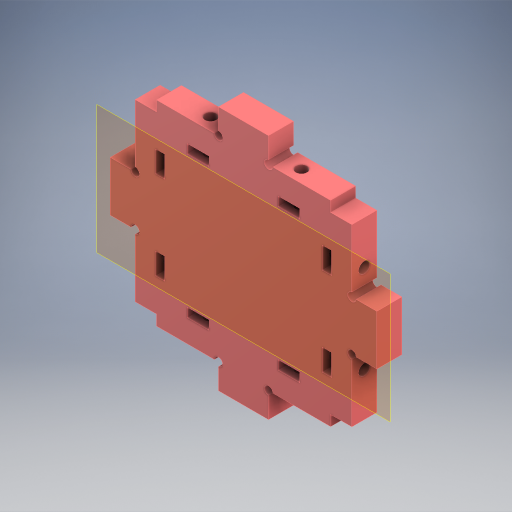
# Autodesk Inventor part: connection_leg_ver2
Saved by Autodesk Inventor 2024 (Build 280153000, 153)
## iProperties
Created: 2024-09-05
Part Number: connection_leg_ver2
Material: PMMA 플라스틱
Document SubType Name: Modeling
Designer: msi
Density: 1.188 g/cm^3
Appearance: 매끄러움 - 빨간색
Author: msi
Autodesk Inventor part; units mm, degrees
ref_plane "YZ Plane" through (0, 0, 0) normal (1, 0, 0) x (0, 1, 0)
ref_plane "XZ Plane" through (0, 0, 0) normal (0, 1, 0) x (-1, 0, 0)
ref_plane "XY Plane" through (0, 0, 0) normal (0, 0, 1) x (1, 0, 0)
ref_plane "작업 평면1" through (0, 0, 0) normal (0, 0, 1) x (1, 0, 0)
sketch "스케치1" plane through (0, 0, 0) normal (0, 0, 1) x (1, 0, 0)
  line L0 (-18.9, 5.4) -> (-21.1, 5.4) projected
  line L1 (-21.1, 5.4) -> (-21.1, 10.6) projected
  line L2 (-21.1, 10.6) -> (-18.9, 10.6) projected
  line L3 (-18.9, 10.6) -> (-18.9, 5.4) projected
  line L4 (-21.1, -5.4) -> (-18.9, -5.4) projected
  line L5 (-18.9, -5.4) -> (-18.9, -10.6) projected
  line L6 (-18.9, -10.6) -> (-21.1, -10.6) projected
  line L7 (-21.1, -10.6) -> (-21.1, -5.4) projected
  line L8 (21.1, 5.4) -> (18.9, 5.4) projected
  line L9 (18.9, 5.4) -> (18.9, 10.6) projected
  line L10 (18.9, 10.6) -> (21.1, 10.6) projected
  line L11 (21.1, 10.6) -> (21.1, 5.4) projected
  line L12 (18.9, -10.6) -> (18.9, -5.4) projected
  line L13 (18.9, -5.4) -> (21.1, -5.4) projected
  line L14 (21.1, -5.4) -> (21.1, -10.6) projected
  line L15 (21.1, -10.6) -> (18.9, -10.6) projected
  circle A0 centre (8, -8) radius 1.35 projected
  circle A1 centre (-8, 8) radius 1.35 projected
  circle A2 centre (-8, -8) radius 1.35 projected
  circle A3 centre (8, 8) radius 1.35 projected
  line L16 (-26, 14) -> (-26, 3) projected
  line L17 (-26, 3) -> (-32, 3) projected
  line L18 (-32, 3) -> (-32, -3) projected
  line L19 (-32, -3) -> (-26, -3) projected
  line L20 (-26, -3) -> (-26, -14) projected
  line L21 (-26, -14) -> (26, -14) projected
  line L22 (26, -14) -> (26, -3) projected
  line L23 (26, -3) -> (32, -3) projected
  line L24 (32, -3) -> (32, 3) projected
  line L25 (32, 3) -> (26, 3) projected
  line L26 (26, 3) -> (26, 14) projected
  line L27 (26, 14) -> (-26, 14) projected
  line L28 (-11, -15.5) -> (-5, -15.5) projected
  line L29 (-5, -15.5) -> (-5, -18.5) projected
  line L30 (-5, -18.5) -> (-11, -18.5) projected
  line L31 (-11, -18.5) -> (-11, -15.5) projected
  line L32 (-5, 15.5) -> (-11, 15.5) projected
  line L33 (-11, 15.5) -> (-11, 18.5) projected
  line L34 (-11, 18.5) -> (-5, 18.5) projected
  line L35 (-5, 18.5) -> (-5, 15.5) projected
  line L36 (11, -18.5) -> (5, -18.5) projected
  line L37 (5, -18.5) -> (5, -15.5) projected
  line L38 (5, -15.5) -> (11, -15.5) projected
  line L39 (11, -15.5) -> (11, -18.5) projected
  line L40 (11, 15.0547) -> (5, 15.0547) projected
  line L41 (5, 15.0547) -> (5, 18.0547) projected
  line L42 (5, 18.0547) -> (11, 18.0547) projected
  line L43 (11, 18.0547) -> (11, 15.0547) projected
  circle A4 centre (8, 8) radius 1.35 projected
  circle A5 centre (-8, -8) radius 1.35 projected
  circle A6 centre (-8, 8) radius 1.35 projected
  circle A7 centre (8, -8) radius 1.35 projected
  line L44 (13.9, 23.5) -> (3, 23.5) projected
  line L45 (3, 23.5) -> (3, 29.5) projected
  line L46 (3, 29.5) -> (-3, 29.5) projected
  line L47 (-3, 29.5) -> (-3, 23.5) projected
  line L48 (-3, 23.5) -> (-13.9, 23.5) projected
  line L49 (-13.9, 23.5) -> (-13.9, -23.5) projected
  line L50 (-13.9, -23.5) -> (-3, -23.5) projected
  line L51 (-3, -23.5) -> (-3, -29.5) projected
  line L52 (-3, -29.5) -> (3, -29.5) projected
  line L53 (3, -29.5) -> (3, -23.5) projected
  line L54 (3, -23.5) -> (13.9, -23.5) projected
  line L55 (13.9, -23.5) -> (13.9, 23.5) projected
  line L56 (13.9, 23.5) -> (-13.9, 23.5)
  line L57 (-13.9, -23.5) -> (13.9, -23.5)
  line L58 (-26, 14) -> (-26, -14)
  line L59 (26, -14) -> (26, 14)
  line L60 (-26, -14) -> (-26, -21)
  line L61 (26, -21) -> (26, -14)
  line L62 (26, 14) -> (26, 21)
  line L63 (-26, 21) -> (-26, 14)
  line L64 (13.9, -23.5) -> (20.9, -23.5)
  line L65 (20.9, 23.5) -> (13.9, 23.5)
  line L66 (-13.9, 23.5) -> (-20.9, 23.5)
  line L67 (-20.9, -23.5) -> (-13.9, -23.5)
  line L68 (26, 21) -> (20.9, 21)
  line L69 (-20.9, 21) -> (-26, 21)
  line L70 (-20.9, -21) -> (-20.9, -23.5)
  line L71 (-20.9, 23.5) -> (-20.9, 21)
  line L72 (20.9, -23.5) -> (20.9, -21)
  line L73 (20.9, 21) -> (20.9, 23.5)
  line L74 (-26, -21) -> (-20.9, -21)
  line L75 (20.9, -21) -> (26, -21)
  line L76 (26, -5.994) -> (26, 6.006)
  line L77 (6, -23.5) -> (-6, -23.5)
  line L78 (-6, -23.5) -> (-6, -29.5)
  line L79 (-6, -29.5) -> (6, -29.5)
  line L80 (6, -29.5) -> (6, -23.5)
  line L81 (6, 23.5) -> (-6, 23.5)
  line L82 (-6, 23.5) -> (-6, 29.5)
  line L83 (-6, 29.5) -> (6, 29.5)
  line L84 (6, 29.5) -> (6, 23.5)
  line L85 (-26, 6) -> (-32, 6)
  line L86 (-32, 6) -> (-32, -6)
  line L87 (-32, -6) -> (-26, -6)
  line L88 (-26, -6) -> (-26, 6)
  line L89 (13.5, 18.1) -> (8.3, 18.1)
  line L90 (8.3, 18.1) -> (8.3, 15.9)
  line L91 (8.3, 15.9) -> (13.5, 15.9)
  line L92 (13.5, 15.9) -> (13.5, 18.1)
  line L93 (13.5, 18.1) -> (8.3, 15.9) construction
  line L94 (8.3, 18.1) -> (13.5, 15.9) construction
  line L95 (-13.5, 18.1) -> (-8.3, 18.1)
  line L96 (-8.3, 18.1) -> (-8.3, 15.9)
  line L97 (-8.3, 15.9) -> (-13.5, 15.9)
  line L98 (-13.5, 15.9) -> (-13.5, 18.1)
  line L99 (-13.5, 18.1) -> (-8.3, 15.9) construction
  line L100 (-8.3, 18.1) -> (-13.5, 15.9) construction
  line L101 (-13.5, -18.1) -> (-8.3, -18.1)
  line L102 (-8.3, -18.1) -> (-8.3, -15.9)
  line L103 (-8.3, -15.9) -> (-13.5, -15.9)
  line L104 (-13.5, -15.9) -> (-13.5, -18.1)
  line L105 (-13.5, -18.1) -> (-8.3, -15.9) construction
  line L106 (-8.3, -18.1) -> (-13.5, -15.9) construction
  line L107 (13.5, -15.9) -> (8.3, -15.9)
  line L108 (8.3, -15.9) -> (8.3, -18.1)
  line L109 (8.3, -18.1) -> (13.5, -18.1)
  line L110 (13.5, -18.1) -> (13.5, -15.9)
  line L111 (13.5, -15.9) -> (8.3, -18.1) construction
  line L112 (8.3, -15.9) -> (13.5, -18.1) construction
  line L113 (-21.1, -8) -> (-18.9, -8)
  line L114 (-18.9, -8) -> (-18.9, -13.2)
  line L115 (-18.9, -13.2) -> (-21.1, -13.2)
  line L116 (-21.1, -13.2) -> (-21.1, -8)
  line L117 (-21.1, -8) -> (-18.9, -13.2) construction
  line L118 (-18.9, -8) -> (-21.1, -13.2) construction
  line L119 (-21.1, 13.2) -> (-18.9, 13.2)
  line L120 (-18.9, 13.2) -> (-18.9, 8)
  line L121 (-18.9, 8) -> (-21.1, 8)
  line L122 (-21.1, 8) -> (-21.1, 13.2)
  line L123 (-21.1, 13.2) -> (-18.9, 8) construction
  line L124 (-18.9, 13.2) -> (-21.1, 8) construction
  line L125 (26, -5.994) -> (26, 6.006)
  line L126 (26, 6) -> (32, 6)
  line L127 (32, 6) -> (32, -6)
  line L128 (32, -6) -> (26, -6)
  line L129 (26, -6) -> (26, 6)
  line L130 (18.9, -8) -> (21.1, -8)
  line L131 (21.1, -8) -> (21.1, -13.2)
  line L132 (21.1, -13.2) -> (18.9, -13.2)
  line L133 (18.9, -13.2) -> (18.9, -8)
  line L134 (18.9, -8) -> (21.1, -13.2) construction
  line L135 (21.1, -8) -> (18.9, -13.2) construction
  line L136 (18.9, 13.2) -> (21.1, 13.2)
  line L137 (21.1, 13.2) -> (21.1, 8)
  line L138 (21.1, 8) -> (18.9, 8)
  line L139 (18.9, 8) -> (18.9, 13.2)
  line L140 (18.9, 13.2) -> (21.1, 8) construction
  line L141 (21.1, 13.2) -> (18.9, 8) construction
  point P0 (0, 0)
  point P1 (10.9, 17)
  point P2 (-10.9, 17)
  point P3 (-10.9, -17)
  point P4 (10.9, -17)
  point P5 (-20, -10.6)
  point P6 (-20, 10.6)
  point P7 (8.3, 18.0547)
  point P8 (11, 15.9)
  point P9 (-13.9, -14)
  point P10 (13.9, -14)
  point P11 (20, -10.6)
  point P12 (20, 10.6)
  dimension "d0" = 7
  dimension "d1" = 7
  dimension "d2" = 7
  dimension "d5" = 12
  dimension "d6" = 6
  dimension "d7" = 12
  dimension "d8" = 6
  dimension "d9" = 12
  dimension "d31" = 5.2
  dimension "d33" = 5.2
  dimension "d34" = 2.2
  dimension "d35" = 5.2
  dimension "d36" = 2.2
  dimension "d37" = 5.2
  dimension "d38" = 2.2
  dimension "d41" = 2.2
  dimension "d42" = 5.2
  dimension "d44" = 2.2
  dimension "d45" = 5.2
  dimension "d69" = 12
  dimension "d70" = 5.2
  dimension "d71" = 2.2
  dimension "d72" = 5.2
  constraints: 172 end point, 30 parallel, 20 midpoint, 16 perpendicular, 15 horizontal, 9 point on line
  measures "d0" distance of L60.end L60.start
  measures "d1" distance of L62.end L62.start
  measures "d2" distance of L65.end L65.start
  measures "d5" distance of L79.end L78.end
  measures "d6" distance of L78.end L77.end
  measures "d7" distance of L82.end L83.end
  measures "d8" distance of L81.end L82.end
  measures "d9" distance of L86.end L85.end
  measures "d31" distance of L91.end L90.end
  measures "d33" distance of L96.end L97.end
  measures "d34" distance of L95.end L96.end
  measures "d35" distance of L103.end L102.end
  measures "d36" distance of L102.end L101.end
  measures "d37" distance of L109.end L108.end
  measures "d38" distance of L108.end L107.end
  measures "d41" distance of L114.end L115.end
  measures "d42" distance of L113.end L114.end
  measures "d44" distance of L120.end L121.end
  measures "d45" distance of L119.end L120.end
  measures "d69" distance of L126.end L127.end
  measures "d70" distance of L130.end L131.end
  measures "d71" distance of L137.end L138.end
  measures "d72" distance of L136.end L137.end
extrude "돌출9" add sketch "스케치1" against normal blind 6 contours L0 L1 L121 L3 | L4 L5 L113 L7 | L8 L9 L138 L11 | L12 L13 L14 L130 | A0 | A1 | A2 | A3 | L27 L49 L21 L20 L58 L16 | L63 L69 L71 L66 L49 L27 | L16 L17 L86 L85 | L49 L48 L56 L44 L55 L27 | L27 L55 L21 L49 | L58 L19 L18 L17 | L55 L65 L73 L68 L62 L27 | L27 L26 L59 L22 L21 L55 | L49 L67 L70 L74 L60 L21 | L21 L55 L54 L57 L50 L49 | L20 L87 L86 L19 | L21 L61 L75 L72 L64 L55 | L82 L83 L47 L48 | L44 L45 L83 L84 | L47 L46 L45 L56 | L50 L51 L79 L78 | L126 L127 L25 L26 | L22 L23 L127 L128 | L80 L79 L53 L54 | L57 L53 L52 L51 | L25 L24 L23 L59 | L28 L29 L30 L31 L101 L102 L103 | L32 L33 L97 L96 L95 L34 L35 | L36 L37 L38 L39 L107 L108 L109 | L40 L41 L42 L90 L91 L43
sketch "스케치7" plane through (-32, -6, 0) normal (-1, 0, 0) x (0, 0, 1)
  line L0 (0, 19.2) -> (0, 14)
  circle A0 centre (-3, 16.6) radius 1.35
  line L1 (0, -2) -> (0, -7.2)
  circle A1 centre (-3, -4.6) radius 1.35
  point P0 (0, 6)
  dimension "d75" = 2.7
  dimension "d76" = 2.7
  constraints: 4 end point, 2 centre point, 2 vertical
  measures "d75" diameter of A0
  measures "d76" diameter of A1
extrude "돌출10" cut sketch "스케치7" against normal blind 16
sketch "스케치8" plane through (32, -6, 0) normal (1, 0, 0) x (0, 0, -1)
  line L0 (6, 19.2) -> (6, 14)
  line L1 (6, -2) -> (6, -7.2)
  circle A0 centre (3, 16.6) radius 1.35
  circle A1 centre (3, -4.6) radius 1.35
  point P0 (0, 6)
  dimension "d79" = 2.7
  dimension "d80" = 2.7
  constraints: 4 end point, 2 centre point, 2 vertical
  measures "d79" diameter of A0
  measures "d80" diameter of A1
extrude "돌출11" cut sketch "스케치8" against normal blind 16
sketch "스케치9" plane through (-6, -29.5, 0) normal (0, -1, 0) x (1, 0, 0)
  line L0 (19.5, -6) -> (14.3, -6)
  line L1 (-2.3, -6) -> (-7.5, -6)
  circle A0 centre (16.9, -3) radius 1.35
  circle A1 centre (-4.9, -3) radius 1.35
  point P0 (6, 0)
  dimension "d83" = 2.7
  dimension "d84" = 2.7
  constraints: 4 end point, 2 centre point, 2 horizontal
  measures "d83" diameter of A0
  measures "d84" diameter of A1
extrude "돌출12" cut sketch "스케치9" against normal blind 16
sketch "스케치10" plane through (-6, 29.5, 0) normal (0, 1, 0) x (1, 0, 0)
  line L0 (19.5, 0) -> (14.3, 0)
  line L1 (-2.3, 0) -> (-7.5, 0)
  circle A0 centre (-4.9, 3) radius 1.35
  circle A1 centre (16.9, 3) radius 1.35
  point P0 (6, 0)
  dimension "d87" = 2.7
  dimension "d88" = 2.7
  constraints: 4 end point, 2 centre point, 2 horizontal
  measures "d87" diameter of A0
  measures "d88" diameter of A1
extrude "돌출13" cut sketch "스케치10" against normal blind 16
sketch "스케치11" plane through (0, 0, 0) normal (0, 0, 1) x (1, 0, 0)
  line L0 (-6, -29.5) -> (6, -29.5) projected
  line L1 (6, -29.5) -> (6, -23.5) projected
  line L2 (6, -23.5) -> (20.9, -23.5) projected
  line L3 (20.9, -23.5) -> (20.9, -21) projected
  line L4 (20.9, -21) -> (26, -21) projected
  line L5 (26, -21) -> (26, -6) projected
  line L6 (26, -6) -> (32, -6) projected
  line L7 (32, -6) -> (32, 6) projected
  line L8 (32, 6) -> (26, 6) projected
  line L9 (26, 6) -> (26, 21) projected
  line L10 (26, 21) -> (20.9, 21) projected
  line L11 (20.9, 21) -> (20.9, 23.5) projected
  line L12 (20.9, 23.5) -> (6, 23.5) projected
  line L13 (6, 23.5) -> (6, 29.5) projected
  line L14 (6, 29.5) -> (-6, 29.5) projected
  line L15 (-6, 29.5) -> (-6, 23.5) projected
  line L16 (-6, 23.5) -> (-20.9, 23.5) projected
  line L17 (-20.9, 23.5) -> (-20.9, 21) projected
  line L18 (-20.9, 21) -> (-26, 21) projected
  line L19 (-26, 21) -> (-26, 6) projected
  line L20 (-26, 6) -> (-32, 6) projected
  line L21 (-32, 6) -> (-32, -6) projected
  line L22 (-32, -6) -> (-26, -6) projected
  line L23 (-26, -6) -> (-26, -21) projected
  line L24 (-26, -21) -> (-20.9, -21) projected
  line L25 (-20.9, -21) -> (-20.9, -23.5) projected
  line L26 (-20.9, -23.5) -> (-6, -23.5) projected
  line L27 (-6, -23.5) -> (-6, -29.5) projected
  line L28 (8.3, -15.9) -> (13.5, -15.9) projected
  line L29 (13.5, -15.9) -> (13.5, -18.1) projected
  line L30 (13.5, -18.1) -> (8.3, -18.1) projected
  line L31 (8.3, -18.1) -> (8.3, -15.9) projected
  line L32 (-8.3, -18.1) -> (-13.5, -18.1) projected
  line L33 (-13.5, -18.1) -> (-13.5, -15.9) projected
  line L34 (-13.5, -15.9) -> (-8.3, -15.9) projected
  line L35 (-8.3, -15.9) -> (-8.3, -18.1) projected
  line L36 (-18.9, -8) -> (-18.9, -13.2) projected
  line L37 (-18.9, -13.2) -> (-21.1, -13.2) projected
  line L38 (-21.1, -13.2) -> (-21.1, -8) projected
  line L39 (-21.1, -8) -> (-18.9, -8) projected
  line L40 (-21.1, 8) -> (-21.1, 13.2) projected
  line L41 (-21.1, 13.2) -> (-18.9, 13.2) projected
  line L42 (-18.9, 13.2) -> (-18.9, 8) projected
  line L43 (-18.9, 8) -> (-21.1, 8) projected
  line L44 (-8.3, 15.9) -> (-13.5, 15.9) projected
  line L45 (-13.5, 15.9) -> (-13.5, 18.1) projected
  line L46 (-13.5, 18.1) -> (-8.3, 18.1) projected
  line L47 (-8.3, 18.1) -> (-8.3, 15.9) projected
  line L48 (8.3, 15.9) -> (8.3, 18.1) projected
  line L49 (8.3, 18.1) -> (13.5, 18.1) projected
  line L50 (13.5, 18.1) -> (13.5, 15.9) projected
  line L51 (13.5, 15.9) -> (8.3, 15.9) projected
  line L52 (18.9, 8) -> (18.9, 13.2) projected
  line L53 (18.9, 13.2) -> (21.1, 13.2) projected
  line L54 (21.1, 13.2) -> (21.1, 8) projected
  line L55 (21.1, 8) -> (18.9, 8) projected
  line L56 (21.1, -8) -> (21.1, -13.2) projected
  line L57 (21.1, -13.2) -> (18.9, -13.2) projected
  line L58 (18.9, -13.2) -> (18.9, -8) projected
  line L59 (18.9, -8) -> (21.1, -8) projected
  circle A0 centre (26, 6) radius 1
  circle A1 centre (26, -6) radius 1
  circle A2 centre (6, -23.5) radius 1
  circle A3 centre (-6, -23.5) radius 1
  circle A4 centre (-26, -6) radius 1
  circle A5 centre (-26, 6) radius 1
  circle A6 centre (-6, 23.5) radius 1
  circle A7 centre (6, 23.5) radius 1
  point P0 (0, 0)
  dimension "d91" = 2
  dimension "d92" = 2
  dimension "d93" = 2
  dimension "d94" = 2
  dimension "d95" = 2
  dimension "d96" = 2
  dimension "d97" = 2
  dimension "d98" = 2
  constraints: 8 centre point, 8 coincident
  measures "d91" diameter of A0
  measures "d92" diameter of A1
  measures "d93" diameter of A2
  measures "d94" diameter of A3
  measures "d95" diameter of A4
  measures "d96" diameter of A5
  measures "d97" diameter of A6
  measures "d98" diameter of A7
extrude "돌출14" cut sketch "스케치11" against normal blind 10 contours A3 L26 L27 | L27 L26 A3 | A2 L2 L1 | L1 L2 A2 | A4 L22 L23 | L23 L22 A4 | A1 L6 L5 | L5 L6 A1 | A5 L19 L20 | L20 L19 A5 | A0 L9 L8 | L8 L9 A0 | A6 L15 L16 | L16 L15 A6 | A7 L13 L12 | L12 L13 A7
